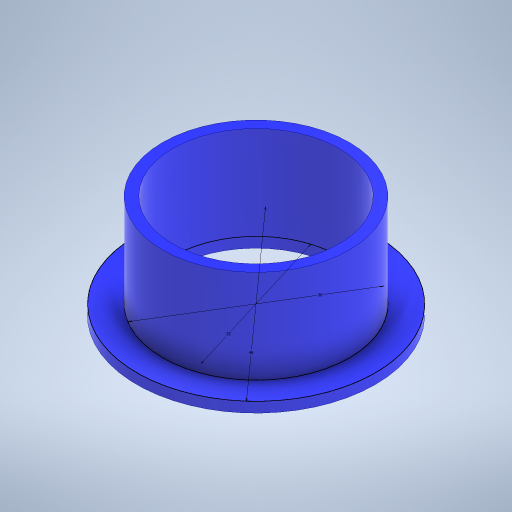
# Autodesk Inventor part: bush
Saved by Autodesk Inventor 2023 (Build 270158000, 158)
## iProperties
Created: 2022-11-04
Part Number: bush
Material: 一般
Document SubType Name: Modeling
Designer: ellie
Density: 1 g/cm^3
Appearance: 青 - 壁塗料 - 光沢
Author: ellie
Autodesk Inventor part; units mm, degrees
ref_plane "YZ Plane" through (0, 0, 0) normal (1, 0, 0) x (0, 1, 0)
ref_plane "XZ Plane" through (0, 0, 0) normal (0, 1, 0) x (-1, 0, 0)
ref_plane "XY Plane" through (0, 0, 0) normal (0, 0, 1) x (1, 0, 0)
sketch "スケッチ1" plane through (0, 0, 0) normal (0, 1, 0) x (-1, 0, 0)
  circle A0 centre (0, 0) radius 18
  circle A1 centre (0, 0) radius 16
  circle A2 centre (0, 0) radius 23
  dimension "d0" = 36
  dimension "d1" = 32
  dimension "d2" = 46
  constraints: 3 centre point, 3 coincident
  measures "d0" diameter of A0
  measures "d1" diameter of A1
  measures "d2" diameter of A2
extrude "押し出し1" add sketch "スケッチ1" along normal blind 18 contours A0
extrude "押し出し2" add sketch "スケッチ1" against normal blind 2 contours A0 | A2
